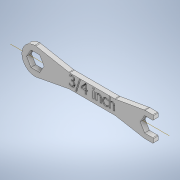
# Autodesk Inventor part: 3_4_inchWrenchV04
Saved by Autodesk Inventor 2020.3 (Build 243373000, 373)
## iProperties
Created: 2019-11-16
Part Number: 3_4_inchWrenchV04
Material: Generic
Document SubType Name: Modeling
Designer: steele
Density: 1 g/cm^3
Appearance: Default
Author: steele
Autodesk Inventor part; units mm, degrees
ref_plane "YZ Plane" through (0, 0, 0) normal (1, 0, 0) x (0, 1, 0)
ref_plane "XZ Plane" through (0, 0, 0) normal (0, 1, 0) x (-1, 0, 0)
ref_plane "XY Plane" through (0, 0, 0) normal (0, 0, 1) x (1, 0, 0)
sketch "Sketch2" plane through (0, 0, 0) normal (0, 0, 1) x (1, 0, 0)
  line L0 (-64.4682, 0) -> (-70.3341, -10.16)
  line L1 (-70.3341, -10.16) -> (-82.0659, -10.16)
  line L2 (-82.0659, -10.16) -> (-87.9318, 0)
  line L3 (-87.9318, 0) -> (-82.0659, 10.16)
  line L4 (-82.0659, 10.16) -> (-70.3341, 10.16)
  line L5 (-70.3341, 10.16) -> (-64.4682, 0)
  line L6 (-76.2, 0) -> (76.2, 0) construction
  line L7 (82.0659, -10.16) -> (70.3341, -10.16)
  line L8 (70.3341, -10.16) -> (64.4682, 0)
  line L9 (64.4682, 0) -> (70.3341, 10.16)
  line L10 (70.3341, 10.16) -> (82.0659, 10.16)
  line L11 (82.0659, 10.16) -> (82.4325, 9.525)
  line L12 (-132.627, 0) -> (135.7899, 0) projected
  line L13 (0, 0) -> (0, 37.2208) construction
  line L14 (0, 9.525) -> (30.7487, 9.525)
  line L15 (0, 9.525) -> (-30.7487, 9.525)
  circle A0 centre (-76.2, 0) radius 18.0818
  line L16 (-87.9318, 0) -> (-94.2818, 0) construction
  arc A1 (61.0244, 14.8673) -> (61.0244, -14.8673) centre (76.2, 0) ccw
  line L17 (87.9318, 0) -> (97.4446, 0) construction
  line L18 (87.9318, 0) -> (89.9839, -16.166) construction
  line L19 (30.7487, 9.525) -> (70.3341, 16.51)
  line L20 (-76.2, 18.0818) -> (-30.7487, 9.525)
  line L21 (70.3341, 10.16) -> (70.3341, 16.51) construction
  line L22 (82.0659, 10.16) -> (82.0659, 16.51)
  line L23 (82.0659, -10.16) -> (82.0659, -16.51)
  line L24 (0, -9.525) -> (30.7487, -9.525)
  line L25 (0, -9.525) -> (-30.7487, -9.525)
  line L26 (30.7487, -9.525) -> (70.3341, -16.51)
  line L27 (-76.2, -18.0818) -> (-30.7487, -9.525)
  line L28 (70.3341, 16.51) -> (82.0659, 16.51)
  line L29 (70.3341, -10.16) -> (70.3341, -16.51) construction
  line L30 (70.3341, -16.51) -> (82.0659, -16.51)
  point P0 (82.0659, 18.5801)
  point P1 (82.0659, -18.5801)
  dimension "centerToBoxEndWrench" = 76.2
  dimension "boltPrintedSize" = 20.32
  dimension "centerToOpenEndWrench" = 76.2
  dimension "d23" = 9.525
  dimension "d24" = 6.35
  dimension "d26" = 6.35
  constraints: 60 end point, 6 point on line, 5 horizontal, 5 symmetric about line, 4 point on circle, 4 vertical, 3 coincident, 3 collinear, 2 centre point, 2 perpendicular, 24 other
  measures "centerToBoxEndWrench" distance of L6.start L13.start
  measures "boltPrintedSize" distance between parallel lines of L1 L4
  measures "centerToOpenEndWrench" distance of L6.end L13.start
  measures "d23" distance between parallel lines of L14 L12
  measures "d24" distance of L16.end L2.end
  measures "d26" distance of L19.end L9.end
extrude "Extrusion2" add sketch "Sketch2" along normal mid plane 6.35 contours L12 A0 L27 L2 L1 L0 | L5 L4 L3 L12 A0 L20 | A0 L20 L15 L14 L19 A1 L12 | L12 A1 L26 L24 L25 L27 A0 | A1 L19 L28 L22 L10 L9 L12 | L12 L8 L7 L23 L30 L26 A1
fillet "Fillet1" radius 0.7937 4 edges at (82.0659, 16.51, 0) (82.0659, 10.16, 0) (82.0659, -10.16, 0) (82.0659, -16.51, 0)
fillet "Fillet2" radius 6.35 8 edges at (-30.7487, -9.525, 0) (30.7487, -9.525, 0) (70.3341, -16.51, 0) (-76.2, -18.0818, 0) (-76.2, 18.0818, 0) (-30.7487, 9.525, 0) (30.7487, 9.525, 0) (70.3341, 16.51, 0)
sketch "Sketch3" plane through (0, 0, 3.175) normal (0, 0, 1) x (1, 0, 0)
  line L0 (-64.4682, 0) -> (64.4682, 0) construction
  spline S0 degree 2 poles (-27.0055, 6.7334) (-27.4686, 6.7334) (-28.3846, 6.5069) (-28.8271, 6.332) knots 0 0 0 1 2 2 2
  spline S1 degree 2 poles (-28.8271, 6.332) (-29.2388, 6.157) (-29.846, 5.7865) (-30.0827, 5.6219) knots 0 0 0 1 2 2 2
  line L1 (-30.0827, 5.6219) -> (-30.1857, 5.6219)
  line L2 (-30.1857, 5.6219) -> (-30.1857, 7.4229)
  spline S2 degree 2 poles (-30.1857, 7.4229) (-29.6299, 7.7214) (-27.7259, 8.2051) (-26.8717, 8.2051) knots 0 0 0 1 2 2 2
  spline S3 degree 2 poles (-26.8717, 8.2051) (-26.0072, 8.2051) (-24.7207, 7.8552) (-24.1959, 7.4847) knots 0 0 0 1 2 2 2
  spline S4 degree 2 poles (-24.1959, 7.4847) (-23.6401, 7.0833) (-23.0638, 5.9203) (-23.0638, 5.1381) knots 0 0 0 1 2 2 2
  spline S5 degree 2 poles (-23.0638, 5.1381) (-23.0638, 4.0884) (-24.4429, 2.5035) (-25.4103, 2.2976) knots 0 0 0 1 2 2 2
  line L3 (-25.4103, 2.2976) -> (-25.4103, 2.1741)
  spline S6 degree 2 poles (-25.4103, 2.1741) (-25.0089, 2.0918) (-24.0929, 1.7213) (-23.7019, 1.3508) knots 0 0 0 1 2 2 2
  spline S7 degree 2 poles (-23.7019, 1.3508) (-23.3108, 0.9906) (-22.8168, -0.1621) (-22.8168, -0.9957) knots 0 0 0 1 2 2 2
  spline S8 degree 2 poles (-22.8168, -0.9957) (-22.8168, -1.8499) (-23.4034, -3.3011) (-23.9386, -3.8568) knots 0 0 0 1 2 2 2
  spline S9 degree 2 poles (-23.9386, -3.8568) (-24.4943, -4.4332) (-26.069, -5.0301) (-27.0673, -5.0301) knots 0 0 0 1 2 2 2
  spline S10 degree 2 poles (-27.0673, -5.0301) (-28.0244, -5.0301) (-29.8975, -4.567) (-30.5356, -4.2479) knots 0 0 0 1 2 2 2
  line L4 (-30.5356, -4.2479) -> (-30.5356, -2.4469)
  line L5 (-30.5356, -2.4469) -> (-30.4121, -2.4469)
  spline S11 degree 2 poles (-30.4121, -2.4469) (-29.8769, -2.8379) (-28.0656, -3.5584) (-27.1702, -3.5584) knots 0 0 0 1 2 2 2
  spline S12 degree 2 poles (-27.1702, -3.5584) (-26.6453, -3.5584) (-25.5955, -3.229) (-25.2456, -2.8482) knots 0 0 0 1 2 2 2
  spline S13 degree 2 poles (-25.2456, -2.8482) (-24.906, -2.4674) (-24.5458, -1.5618) (-24.5458, -0.8722) knots 0 0 0 1 2 2 2
  spline S14 degree 2 poles (-24.5458, -0.8722) (-24.5458, -0.1827) (-24.9472, 0.7127) (-25.3074, 0.97) knots 0 0 0 1 2 2 2
  spline S15 degree 2 poles (-25.3074, 0.97) (-25.6676, 1.2273) (-26.6453, 1.4228) (-27.2216, 1.4228) knots 0 0 0 1 2 2 2
  line L6 (-27.2216, 1.4228) -> (-27.9421, 1.4228)
  line L7 (-27.9421, 1.4228) -> (-27.9421, 2.8328)
  line L8 (-27.9421, 2.8328) -> (-27.376, 2.8328)
  spline S16 degree 2 poles (-27.376, 2.8328) (-26.2336, 2.8328) (-24.7928, 3.9237) (-24.7928, 4.9632) knots 0 0 0 1 2 2 2
  spline S17 degree 2 poles (-24.7928, 4.9632) (-24.7928, 5.4469) (-25.1633, 6.1364) (-25.4617, 6.3423) knots 0 0 0 1 2 2 2
  spline S18 degree 2 poles (-25.4617, 6.3423) (-25.7808, 6.5584) (-26.563, 6.7334) (-27.0055, 6.7334) knots 0 0 0 1 2 2 2
  line L9 (-15.6229, 8.5035) -> (-20.5938, -7.5207)
  line L10 (-20.5938, -7.5207) -> (-22.0346, -7.5207)
  line L11 (-22.0346, -7.5207) -> (-17.0843, 8.5035)
  line L12 (-17.0843, 8.5035) -> (-15.6229, 8.5035)
  line L13 (-6.0515, -0.3988) -> (-7.5644, -0.3988)
  line L14 (-7.5644, -0.3988) -> (-7.5644, -4.7625)
  line L15 (-7.5644, -4.7625) -> (-9.2008, -4.7625)
  line L16 (-9.2008, -4.7625) -> (-9.2008, -0.3988)
  line L17 (-9.2008, -0.3988) -> (-14.8098, -0.3988)
  line L18 (-14.8098, -0.3988) -> (-14.8098, 1.392)
  line L19 (-14.8098, 1.392) -> (-9.1288, 7.9375)
  line L20 (-9.1288, 7.9375) -> (-7.5644, 7.9375)
  line L21 (-7.5644, 7.9375) -> (-7.5644, 0.97)
  line L22 (-7.5644, 0.97) -> (-6.0515, 0.97)
  line L23 (-6.0515, 0.97) -> (-6.0515, -0.3988)
  line L24 (-9.2008, 0.97) -> (-9.2008, 5.9306)
  line L25 (-9.2008, 5.9306) -> (-13.4719, 0.97)
  line L26 (-13.4719, 0.97) -> (-9.2008, 0.97)
  line L27 (2.6347, -4.7625) -> (1.0292, -4.7625)
  line L28 (1.0292, -4.7625) -> (1.0292, 4.7676)
  line L29 (1.0292, 4.7676) -> (2.6347, 4.7676)
  line L30 (2.6347, 4.7676) -> (2.6347, -4.7625)
  line L31 (2.7479, 6.3526) -> (0.9263, 6.3526)
  line L32 (0.9263, 6.3526) -> (0.9263, 8.0198)
  line L33 (0.9263, 8.0198) -> (2.7479, 8.0198)
  line L34 (2.7479, 8.0198) -> (2.7479, 6.3526)
  line L35 (12.4736, -4.7625) -> (10.8681, -4.7625)
  line L36 (10.8681, -4.7625) -> (10.8681, 0.6715)
  spline S19 degree 2 poles (10.8681, 0.6715) (10.8681, 1.3302) (10.7446, 2.4623) (10.5593, 2.8019) knots 0 0 0 1 2 2 2
  spline S20 degree 2 poles (10.5593, 2.8019) (10.3638, 3.1621) (9.6639, 3.5121) (9.067, 3.5121) knots 0 0 0 1 2 2 2
  spline S21 degree 2 poles (9.067, 3.5121) (8.4701, 3.5121) (7.2042, 2.874) (6.597, 2.3594) knots 0 0 0 1 2 2 2
  line L37 (6.597, 2.3594) -> (6.597, -4.7625)
  line L38 (6.597, -4.7625) -> (4.9915, -4.7625)
  line L39 (4.9915, -4.7625) -> (4.9915, 4.7676)
  line L40 (4.9915, 4.7676) -> (6.597, 4.7676)
  line L41 (6.597, 4.7676) -> (6.597, 3.7076)
  spline S22 degree 2 poles (6.597, 3.7076) (7.3174, 4.356) (8.7068, 5.0352) (9.489, 5.0352) knots 0 0 0 1 2 2 2
  spline S23 degree 2 poles (9.489, 5.0352) (10.8887, 5.0352) (12.4736, 3.1827) (12.4736, 1.4228) knots 0 0 0 1 2 2 2
  line L42 (12.4736, 1.4228) -> (12.4736, -4.7625)
  spline S24 degree 2 poles (18.5148, -4.9786) (17.5268, -4.9786) (15.8904, -4.3714) (15.3038, -3.7539) knots 0 0 0 1 2 2 2
  spline S25 degree 2 poles (15.3038, -3.7539) (14.7172, -3.1467) (14.0688, -1.2736) (14.0688, -0.018) knots 0 0 0 1 2 2 2
  spline S26 degree 2 poles (14.0688, -0.018) (14.0688, 1.2376) (14.7378, 3.0695) (15.3038, 3.687) knots 0 0 0 1 2 2 2
  spline S27 degree 2 poles (15.3038, 3.687) (15.8699, 4.3148) (17.5474, 4.9838) (18.5148, 4.9838) knots 0 0 0 1 2 2 2
  spline S28 degree 2 poles (18.5148, 4.9838) (19.297, 4.9838) (20.7584, 4.5412) (21.3245, 4.2531) knots 0 0 0 1 2 2 2
  line L43 (21.3245, 4.2531) -> (21.3245, 2.452)
  line L44 (21.3245, 2.452) -> (21.2318, 2.452)
  spline S29 degree 2 poles (21.2318, 2.452) (21.0569, 2.5961) (20.5217, 2.9666) (20.1409, 3.1621) knots 0 0 0 1 2 2 2
  spline S30 degree 2 poles (20.1409, 3.1621) (19.8013, 3.3268) (18.8956, 3.5841) (18.484, 3.5841) knots 0 0 0 1 2 2 2
  spline S31 degree 2 poles (18.484, 3.5841) (17.2387, 3.5841) (15.7258, 1.7007) (15.7258, -0.018) knots 0 0 0 1 2 2 2
  spline S32 degree 2 poles (15.7258, -0.018) (15.7258, -1.6956) (17.1872, -3.579) (18.484, -3.579) knots 0 0 0 1 2 2 2
  spline S33 degree 2 poles (18.484, -3.579) (19.2661, -3.579) (20.6864, -2.9306) (21.2318, -2.4263) knots 0 0 0 1 2 2 2
  line L45 (21.2318, -2.4263) -> (21.3245, -2.4263)
  line L46 (21.3245, -2.4263) -> (21.3245, -4.2273)
  spline S34 degree 2 poles (21.3245, -4.2273) (21.0878, -4.3405) (20.3673, -4.6596) (20.0792, -4.7316) knots 0 0 0 1 2 2 2
  spline S35 degree 2 poles (20.0792, -4.7316) (19.6675, -4.8551) (19.0191, -4.9786) (18.5148, -4.9786) knots 0 0 0 1 2 2 2
  line L47 (30.268, -4.7625) -> (28.6625, -4.7625)
  line L48 (28.6625, -4.7625) -> (28.6625, 0.6715)
  spline S36 degree 2 poles (28.6625, 0.6715) (28.6625, 1.3302) (28.539, 2.4623) (28.3537, 2.8019) knots 0 0 0 1 2 2 2
  spline S37 degree 2 poles (28.3537, 2.8019) (28.1582, 3.1621) (27.4583, 3.5121) (26.8614, 3.5121) knots 0 0 0 1 2 2 2
  spline S38 degree 2 poles (26.8614, 3.5121) (26.2645, 3.5121) (24.9986, 2.874) (24.3914, 2.3594) knots 0 0 0 1 2 2 2
  line L49 (24.3914, 2.3594) -> (24.3914, -4.7625)
  line L50 (24.3914, -4.7625) -> (22.7859, -4.7625)
  line L51 (22.7859, -4.7625) -> (22.7859, 8.5035)
  line L52 (22.7859, 8.5035) -> (24.3914, 8.5035)
  line L53 (24.3914, 8.5035) -> (24.3914, 3.7076)
  spline S39 degree 2 poles (24.3914, 3.7076) (25.1118, 4.356) (26.5012, 5.0352) (27.2834, 5.0352) knots 0 0 0 1 2 2 2
  spline S40 degree 2 poles (27.2834, 5.0352) (28.6831, 5.0352) (30.268, 3.1827) (30.268, 1.4228) knots 0 0 0 1 2 2 2
  line L54 (30.268, 1.4228) -> (30.268, -4.7625)
  point P0 (0, 0)
  constraints: 2 end point, 2 horizontal
extrude "Extrusion3" cut sketch "Sketch3" against normal through all
equation "\"centerToBoxEndWrench\" = 4 * boltSize"
equation "\"boltPrintedSize\" = boltSize + boltGap"
equation "\"centerToOpenEndWrench\" = 4 * boltSize"
equation "\"d23\" = 0.5 * boltSize"
equation "\"d24\" = minWallThickness"
equation "\"d26\" = minWallThickness"
equation "\"d27\" = minWallThickness"
equation "\"minWallThickness\" = 6.35"
equation "\"boltGap\" = 1.27"
equation "\"boltSize\" = 19.05"
body "Solid2"
